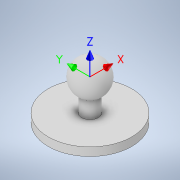
# Autodesk Inventor part: FP
Saved by Autodesk Inventor 2020.1 (Build 241239000, 239)
## iProperties
Created: 2019-10-24
Part Number: FP
Material: Generic
Document SubType Name: Modeling
Designer: sshel
Density: 1 g/cm^3
Appearance: Default
Author: sshel
Autodesk Inventor part; units mm, degrees
ref_plane "YZ Plane" through (0, 0, 0) normal (1, 0, 0) x (0, 1, 0)
ref_plane "XZ Plane" through (0, 0, 0) normal (0, 1, 0) x (-1, 0, 0)
ref_plane "XY Plane" through (0, 0, 0) normal (0, 0, 1) x (1, 0, 0)
sketch "Sketch2" plane through (0, 0, 0) normal (0, 1, 0) x (-1, 0, 0)
  line L0 (0, 143.7774) -> (0, -95.5661) construction
  line L1 (190.8875, 0) -> (-168.3726, 0)
  arc A0 (20, -34.641) -> (0, 40) centre (0, 0) ccw
  line L2 (0, 0) -> (0, -94.641)
  line L3 (0, -94.641) -> (100, -94.641)
  line L4 (100, -94.641) -> (100, -74.641)
  line L5 (100, -74.641) -> (20, -74.641)
  line L6 (20, -74.641) -> (20, -34.641)
  line L7 (0, 0) -> (0, 40)
  dimension "d0" = 40
  dimension "ht" = 40
  dimension "base_thick" = 20
  dimension "base_radius" = 100
  dimension "d11" = 20
  constraints: 16 end point, 5 perpendicular, 3 vertical, 2 point on circle, 1 centre point, 1 coincident, 1 point on line
  measures "d0" radius of A0
  measures "ht" distance of L5.end L6.end
  measures "base_thick" distance of L3.end L4.end
  measures "base_radius" distance of L2.end L3.end
  measures "d11" distance between parallel lines of L2 L6
revolve "Revolution2" add sketch "Sketch2" angle 360 about axis through (0, 0, 143.7774) along (0, 0, -1)
equation "\"d0\" = S_radius"
equation "\"ht\" = 2 * rod_radius"
equation "\"base_thick\" = rod_radius"
equation "\"base_radius\" = 5 * rod_radius"
equation "\"d11\" = rod_radius"
equation "\"rod_radius\" = 20"
equation "\"S_radius\" = 2 * rod_radius"
body "Solid2"
